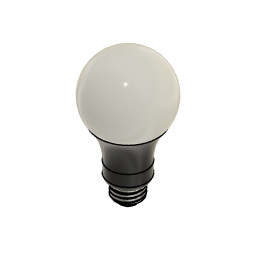
LED Bulb (Autodesk Fusion 360 design; units mm, degrees)
Autodesk Fusion 360 part; units mm, degrees
sketch "Sketch1" plane through (0, 0, 0) normal (0, 0, 1) x (1, 0, 0)
  circle A0 centre (0, 0) radius 15
  dimension "d1" = 30
  constraint coincident A0.centre origin
  measures "d1" diameter of A0
extrude "Extrude1" add sketch "Sketch1" along normal blind 40 makes body 1
sketch "Sketch5" plane through (0, 0, 0) normal (0, 1, 0) x (1, 0, 0)
  line L0 (0, -40) -> (0, -60) construction
  dimension "d22" = 20
  constraint vertical L0
  measures "d22" distance of L0.start L0.end
sphere "SpherePrimitive2" add diameter 61 placed x (1, 0, 0) y (0, 0, -1) z (0, 1, 0) at (0, 0, 60) bodies 1
fillet "Fillet4" radius 45 1 edges at (-13.9849, 5.4242, 33.4435) on bodies 1
fillet "Fillet2" radius 5 1 edges at (-13.9849, -5.4242, 0) on bodies 1
sketch "Sketch3" plane through (0, 0, 0) normal (0, 0, 1) x (1, 0, 0)
  circle A0 centre (0, 0) radius 2.5
  dimension "d10" = 5
  constraint coincident A0.centre origin
  measures "d10" diameter of A0
extrude "Extrude2" add 1 faces at (2.3712, -3.5556, 0) along direction (0, 0, -1) blind 15 separate body on bodies 1 makes body 2
thread "Thread1" "ANSI Metric M Profile 22.0 M22x3 6g" major diameter 21.7645 minor diameter 18.3374 pitch 3 angle 60 modelled right hand crest width 0.4298 on face at (9.9503, -0.9957, -10) from (0, 0, -2) to (0, 0, -12) crest through (10.8823, 0, 0.75) on bodies 2
chamfer "Chamfer1" distance 5 angle 45 1 edges at (-10.1458, 3.9352, -15) on bodies 2
fillet "Fillet3" radius 2 1 edges at (-5.4842, -2.1271, -15) on bodies 2
sketch "Sketch4" plane through (0, 0, -15) normal (0, 0, -1) x (1, 0, 0)
  circle A0 centre (0, 0) radius 5.0538
cylinder "CylinderPrimitive1" add diameter 10.108 height 2 placed x (0, 1, 0) y (1, 0, 0) z (0, 0, -1) at (0, 0, -15) bodies 2
chamfer "Chamfer2" distance 2 angle 45 1 edges at (-1.8276, -4.712, -17) on bodies 2
named bodies: "Light", "Power"
